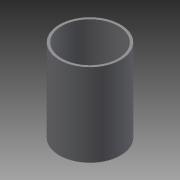
# Autodesk Inventor part: 020.825-FO1_BM_tube
Saved by Autodesk Inventor 2014 SP2 (Build 180246200, 246)
## iProperties
Created: 2020-02-04
Part Number: 020.825-FO1_BM_tube
Material: Generic
Catalog Web Link: www.cadenas.de
Description: FO1_basic_model_tube-Bimba FLAT-1
Vendor: BIMBA
Document SubType Name: Modeling
Designer: psadmin
Manufacturer: BIMBA
Mass: 0.597329 g
Surface Area: 20.1675 cm^2
Volume: 0.597329 cm^3
Density: 1 g/cm^3
Appearance: PSOLRGB-180-180-180
Category: PARTsolutions
Company: BIMBA
Title: 020.825-FO1_BM_tube
Author: Cadenas PARTsolutions
Comments: Bimba FLAT-1
PSOL_IDENT_0: {$CADENAS_DATA\23d-libs\bimba\bimba_brand\bimba_imperial\bimba_full_line\flat_cylinders\fo1\fo1_basi
PSOL_IDENT_1: c_model_tube.prj},207 {VTYP=3D},{NB=020.825-FO1_BM_tube},{LINA=020.825-FO1_BM_tube},{NN=FO1_basic_mo
PSOL_IDENT_2: del_tube},{DATE=22.01.2020 09:06:04},{GEOMDATE=17.09.2018 12:15:13},{VERSION=},{LINEID=10},{WBVAR=ST
PSOL_IDENT_3: ROKE,AB},{WBNUMERIC=STROKE}  {NB=020.825-FO1_BM_tube},{LINA=020.825-FO1_BM_tube},{KT=DUMMY},{PN=020.
PSOL_IDENT_4: 825-FO1_BM_tube},{BORE=0.56250000},{BOREPN=02},{STROKE=0.82500},{STROKEMIN=0.2},{AB=},{A=1.12000000}
PSOL_IDENT_5: ,{BA=0.56000},{BB=0.69000},{BC=0.81},{BD=1.06},{C=0.88000000},{DD=2.00000000},{D=0.11200000},{CPIL=0
PSOL_IDENT_6: .12000000},{DC=0.18800000},{DCP=0.12000000},{DCD=0.85500000},{ES=0.16400000},{EC=0.00000000},{ED=0.4
PSOL_IDENT_7: 6000000},{F=0.25000000},{H=0.22000000},{J=0.34000000},{K=0.14000000},{L=0.19000000},{LDP=0.20000000}
PSOL_IDENT_8: ,{LP=0.16000000},{LPDP=0.28000000},{TD=0.65700000},{TDDP=0.10000},{TD1=0.59500},{TD2=0.61000},{TDIN=
PSOL_IDENT_9: 0.56200},{LSF=0.31250000},{LSFDP=0.02000000},{BC1=0.81000},{BC2=1.38000},{BC3=1.96000},{BC4=2.52000}
PSOL_IDENT_10: ,{BD1=1.06000},{BD2=1.62000},{BD3=2.14000},{BD4=2.70000},{TDAB=0.690},{TDA=0.610},{UNANG=15.000}
NN: FO1_basic_model_tube
NT: Bimba FLAT-1
NB: 020.825-FO1_BM_tube
NBSYN: $PN.
LINA: 020.825-FO1_BM_tube
PN: 020.825-FO1_BM_tube
BORE: 0
BOREPN: 02
STROKE: 0.825
AB: Standard
A: 1.12
BA: 0.56
BB: 0.69
C: 0.88
DD: 2
D: 0.112
CPIL: 0.12
DC: 0.188
DCP: 0.12
DCD: 0.855
ES: 0.164
EC: 0
ED: 0.46
F: 0.25
H: 0.22
J: 0.34
K: 0.14
L: 0.19
LDP: 0.2
LP: 0.16
LPDP: 0.28
TD: 0.657
TDDP: 0.1
TD1: 0.595
TD2: 0.61
TDIN: 0.562
LSF: 0.3125
LSFDP: 0.02
BC1: 0.81
BC2: 1.38
BC3: 1.96
BC4: 2.52
BD1: 1.06
BD2: 1.62
BD3: 2.14
BD4: 2.7
TDAB: 0.69
UNANG: 15
SUPPLIER: BIMBA
ARTICLENO: 020.825-FO1_BM_tube
BOMINFO: 020.825-FO1_BM_tube
CREATOR: CADENAS GmbH
Autodesk Inventor part; units mm, degrees
sketch "Sketch_4" plane through (0, 0, 0) normal (0, 0, 1) x (1, 0, 0)
  line L0 (0, 0) -> (0, 20.955)
  line L1 (7.1374, 20.955) -> (7.1374, 0)
  line L2 (7.1374, 0) -> (7.747, 0)
  line L3 (7.747, 0) -> (7.747, 20.955)
  line L4 (7.747, 20.955) -> (7.1374, 20.955)
  constraints: 10 end point
revolve "Revolution1" add sketch "Sketch_4" angle 360 about axis through (0, 0, 0) along (0, -1, 0)
ref_plane "rod_to_part_XY" through (0, 10.4775, 0) normal (0, 1, 0) x (1, 0, 0)
ref_plane "rod_to_part_YZ" through (0, 10.4775, 0) normal (1, 0, 0) x (0, 0, -1)
ref_plane "rod_to_part_ZX" through (0, 10.4775, 0) normal (0, 0, -1) x (0, 1, 0)
ref_plane "to_road_XY" through (0, 10.4775, 0) normal (0, 1, 0) x (1, 0, 0)
ref_plane "to_road_YZ" through (0, 10.4775, 0) normal (1, 0, 0) x (0, 0, -1)
ref_plane "to_road_ZX" through (0, 10.4775, 0) normal (0, 0, -1) x (0, 1, 0)
ref_plane "track1_XY" through (-7.747, 18.415, 0) normal (0, 1, 0) x (1, 0, 0)
ref_plane "track1_YZ" through (-7.747, 18.415, 0) normal (1, 0, 0) x (0, 0, -1)
ref_plane "track1_ZX" through (-7.747, 18.415, 0) normal (0, 0, -1) x (0, 1, 0)
ref_plane "track1_u_XY" through (-7.747, 2.54, 0) normal (0, 1, 0) x (1, 0, 0)
ref_plane "track1_u_YZ" through (-7.747, 2.54, 0) normal (1, 0, 0) x (0, 0, -1)
ref_plane "track1_u_ZX" through (-7.747, 2.54, 0) normal (0, 0, -1) x (0, 1, 0)
ref_plane "track2_XY" through (0, 18.415, -7.747) normal (0, 1, 0) x (1, 0, 0)
ref_plane "track2_YZ" through (0, 18.415, -7.747) normal (1, 0, 0) x (0, 0, -1)
ref_plane "track2_ZX" through (0, 18.415, -7.747) normal (0, 0, -1) x (0, 1, 0)
ref_plane "track2_u_XY" through (0, 2.54, -7.747) normal (0, 1, 0) x (1, 0, 0)
ref_plane "track2_u_YZ" through (0, 2.54, -7.747) normal (1, 0, 0) x (0, 0, -1)
ref_plane "track2_u_ZX" through (0, 2.54, -7.747) normal (0, 0, -1) x (0, 1, 0)
ref_plane "track3_XY" through (7.747, 18.415, 0) normal (0, 1, 0) x (1, 0, 0)
ref_plane "track3_YZ" through (7.747, 18.415, 0) normal (1, 0, 0) x (0, 0, -1)
ref_plane "track3_ZX" through (7.747, 18.415, 0) normal (0, 0, -1) x (0, 1, 0)
ref_plane "track3_u_XY" through (7.747, 2.54, 0) normal (0, 1, 0) x (1, 0, 0)
ref_plane "track3_u_YZ" through (7.747, 2.54, 0) normal (1, 0, 0) x (0, 0, -1)
ref_plane "track3_u_ZX" through (7.747, 2.54, 0) normal (0, 0, -1) x (0, 1, 0)
ref_plane "track4_XY" through (0, 18.415, 7.747) normal (0, 1, 0) x (1, 0, 0)
ref_plane "track4_YZ" through (0, 18.415, 7.747) normal (1, 0, 0) x (0, 0, -1)
ref_plane "track4_ZX" through (0, 18.415, 7.747) normal (0, 0, -1) x (0, 1, 0)
ref_plane "track4_u_XY" through (0, 2.54, 7.747) normal (0, 1, 0) x (1, 0, 0)
ref_plane "track4_u_YZ" through (0, 2.54, 7.747) normal (1, 0, 0) x (0, 0, -1)
ref_plane "track4_u_ZX" through (0, 2.54, 7.747) normal (0, 0, -1) x (0, 1, 0)
ref_plane "tube_rear_XY" through (0, 20.955, 0) normal (0, 1, 0) x (1, 0, 0)
ref_plane "tube_rear_YZ" through (0, 20.955, 0) normal (1, 0, 0) x (0, 0, -1)
ref_plane "tube_rear_ZX" through (0, 20.955, 0) normal (0, 0, -1) x (0, 1, 0)
ref_plane "tube_rod_guide_XY" through (0, 0, 0) normal (0, 1, 0) x (1, 0, 0)
ref_plane "tube_rod_guide_YZ" through (0, 0, 0) normal (1, 0, 0) x (0, 0, -1)
ref_plane "tube_rod_guide_ZX" through (0, 0, 0) normal (0, 0, -1) x (0, 1, 0)
body "Solid1"
